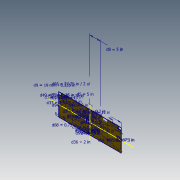
# Autodesk Inventor part: FLUGGER AIR VALVE MTG BRKT
Saved by Autodesk Inventor 2020.3 (Build 243373000, 373)
## iProperties
RuleStatus: InUse
AfterDocSave0: file://Part Number Cleaner
Created: 2019-10-25
Material: ACRYLIC, BLACK
Vendor: HHMI: JRC - ID&F
Document SubType Name: Modeling
Designer: arnoldj
Density: 1 g/cm^3
Appearance: Gold
DESIGN DEPARTMENT: HHMI: JRC - ID&F
ALTERED ITEM PART NUMBER: N/A
ALTERED ITEM VENDOR: N/A
ALTERED ITEM DESCRIPTION: N/A
Author: arnoldj
Revision Number: 0
Autodesk Inventor part; units mm, degrees
ref_plane "YZ Plane" through (0, 0, 0) normal (1, 0, 0) x (0, 1, 0)
ref_plane "XZ Plane" through (0, 0, 0) normal (0, 1, 0) x (-1, 0, 0)
ref_plane "XY Plane" through (0, 0, 0) normal (0, 0, 1) x (1, 0, 0)
sketch "Sketch1" plane through (0, 0, 0) normal (0, 0, 1) x (1, 0, 0)
  line L0 (0, 186.69) -> (0, -186.69) projected
  line L1 (-533.4, 0) -> (533.4, 0) projected
  line L2 (381, -133.35) -> (-381, -133.35)
  line L3 (-381, -133.35) -> (-381, 133.35)
  line L4 (-381, 133.35) -> (381, 133.35)
  line L5 (381, 133.35) -> (381, -133.35)
  line L6 (381, -133.35) -> (-381, 133.35) construction
  line L7 (-381, -133.35) -> (381, 133.35) construction
  line L8 (-170.942, 32.258) -> (-127, 32.258) construction
  line L9 (-127, 32.258) -> (-127, 6.35) construction
  line L10 (-127, 6.35) -> (-170.942, 6.35) construction
  line L11 (-170.942, 6.35) -> (-170.942, 32.258) construction
  line L12 (127, 32.258) -> (170.942, 32.258) construction
  line L13 (170.942, 32.258) -> (170.942, 6.35) construction
  line L14 (170.942, 6.35) -> (127, 6.35) construction
  line L15 (127, 6.35) -> (127, 32.258) construction
  line L16 (-381, 101.6) -> (-346.075, 101.6)
  line L17 (-346.075, 101.6) -> (-346.075, 133.35)
  line L18 (346.075, 133.35) -> (346.075, 101.6)
  line L19 (346.075, 101.6) -> (381, 101.6)
  line L20 (368.3, -114.3) -> (-368.3, -114.3) construction
  line L21 (-368.3, -114.3) -> (-368.3, 82.55) construction
  line L22 (-368.3, 82.55) -> (368.3, 82.55) construction
  line L23 (368.3, 82.55) -> (368.3, -114.3) construction
  line L24 (368.3, -114.3) -> (-368.3, 82.55) construction
  line L25 (-368.3, -114.3) -> (368.3, 82.55) construction
  line L26 (328.6125, -23.8125) -> (357.1875, -23.8125)
  line L27 (357.1875, -23.8125) -> (357.1875, 23.8125)
  line L28 (357.1875, 23.8125) -> (328.6125, 23.8125)
  line L29 (328.6125, 23.8125) -> (328.6125, -23.8125)
  line L30 (328.6125, -23.8125) -> (357.1875, 23.8125) construction
  line L31 (357.1875, -23.8125) -> (328.6125, 23.8125) construction
  line L32 (-42.8625, -23.8125) -> (-14.2875, -23.8125)
  line L33 (-14.2875, -23.8125) -> (-14.2875, 23.8125)
  line L34 (-14.2875, 23.8125) -> (-42.8625, 23.8125)
  line L35 (-42.8625, 23.8125) -> (-42.8625, -23.8125)
  line L36 (-42.8625, -23.8125) -> (-14.2875, 23.8125) construction
  line L37 (-14.2875, -23.8125) -> (-42.8625, 23.8125) construction
  point P0 (0, 0)
  point P1 (-159.004, 6.35)
  point P2 (138.938, 6.35)
  point P3 (-279.4, 122.859)
  point P4 (279.4, 122.859)
  point P5 (-5.08, 122.859)
  point P6 (0, -15.875)
  point P7 (342.9, 0)
  point P8 (-28.575, 0)
  dimension "d0" = 762
  dimension "d1" = 266.7
  dimension "d2" = 43.942
  dimension "d3" = 25.908
  dimension "d4" = 32.004
  dimension "d5" = 127
  dimension "d7" = 32.004
  dimension "d8" = 127
  dimension "d9" = 10.491
  dimension "d65" = 31.75
  dimension "d66" = 346.075
  dimension "d67" = 736.6
  dimension "d68" = 19.05
  dimension "d69" = 19.05
  dimension "d84" = 279.4
  dimension "d85" = 279.4
  dimension "d86" = 5.08
  dimension "d87" = 28.575
  dimension "d88" = 47.625
  dimension "d89" = 0
  dimension "d90" = 28.575
  dimension "d91" = 342.9
  dimension "d94" = 101.092
  constraints: 72 end point, 12 parallel, 10 point on line, 8 coincident, 8 midpoint, 8 perpendicular, 7 horizontal, 5 equal length, 2 horizontal alignment, 1 vertical
  measures "d0" distance of L3.end L4.end
  measures "d1" distance of L2.end L3.end
  measures "d2" distance of L8.start L8.end
  measures "d3" distance of L10.end L8.start
  measures "d4" distance from line of L9 point (-159.004, 6.35)
  measures "d5" distance between parallel lines of L0 L9
  measures "d7" distance from line of L13 point (138.938, 6.35)
  measures "d8" distance between parallel lines of L0 L15
  measures "d9" distance from line of point (-279.4, 122.859) L4
  measures "d65" distance of L16.end L17.end
  measures "d66" distance between parallel lines of L0 L17
  measures "d67" distance of L21.end L22.end
  measures "d68" distance between parallel lines of L20 L2
  measures "d69" distance between parallel lines of L22 L16
  measures "d84" distance from line of L0 point (-279.4, 122.859)
  measures "d85" distance from line of point (279.4, 122.859) L0
  measures "d86" distance from line of L0 point (-5.08, 122.859)
  measures "d87" distance of L33.end L34.end
  measures "d88" distance of L26.end L27.end
  measures "d89" distance from line of point (-28.575, 0) L1
  measures "d90" distance from line of L0 point (-28.575, 0)
  measures "d91" distance from line of point (342.9, 0) L0
  measures "d94" distance from line of point (-170.942, 32.258) L4
extrude "Extrusion1" add sketch "Sketch1" against normal blind 5.842 contours L4 L18 L19 L5 L1 L27 L28 L29 L0 | L0 L1 L33 L34 L35 L3 L16 L17 L4 | L1 L29 L26 L27 L5 L2 L0 | L0 L2 L3 L1 L35 L32 L33 | L33 L32 L35 L1 | L1 L35 L34 L33 | L29 L28 L27 L1 | L1 L27 L26 L29
hole "Hole1" at (-170.942, 32.258, 0) at (-127, 32.258, 0) at (-159.004, 6.35, 0) at (127, 32.258, 0) at (170.942, 32.258, 0) at (138.938, 6.35, 0) direction (0, 0, -1) diameter 3.1242 end through all
thread "Thread1" size "M4x0.7" class "6H" standard "ANSI Metric M Profile" full length
thread "Thread2" size "5-40 UNC" class "2B" standard "ANSI Unified Screw Threads" full length
hole "Hole2" at (-279.4, 122.859, 0) at (279.4, 122.859, 0) at (-5.08, 122.859, 0) direction (0, 0, -1) diameter 6.731 end through all
fillet "Fillet1" radius 9.525 2 edges at (381, -133.35, -2.921) (-381, -133.35, -2.921)
sketch "Sketch2" plane through (0, 0, 0) normal (0, 0, 1) x (1, 0, 0)
  line L0 (0, 118.11) -> (0, -175.26) projected
  line L1 (-520.065, 0) -> (520.065, 0) projected
  line L2 (215.9, -82.55) -> (-215.9, -82.55) construction
  line L3 (-215.9, -82.55) -> (-215.9, 38.1) construction
  line L4 (-215.9, 38.1) -> (215.9, 38.1) construction
  line L5 (215.9, 38.1) -> (215.9, -82.55) construction
  line L6 (215.9, -82.55) -> (-215.9, 38.1) construction
  line L7 (-215.9, -82.55) -> (215.9, 38.1) construction
  line L8 (-371.475, -133.35) -> (371.475, -133.35) construction
  line L9 (-22.86, -121.4084) -> (-22.86, -107.1916) construction
  line L10 (-20.574, -121.4084) -> (-20.574, -107.1916)
  line L11 (-25.146, -107.1916) -> (-25.146, -121.4084)
  arc A0 (-25.146, -121.4084) -> (-20.574, -121.4084) centre (-22.86, -121.4084) ccw
  arc A1 (-20.574, -107.1916) -> (-25.146, -107.1916) centre (-22.86, -107.1916) ccw
  line L12 (-7.62, -121.4084) -> (-7.62, -107.1916) construction
  line L13 (-5.334, -121.4084) -> (-5.334, -107.1916)
  line L14 (-9.906, -107.1916) -> (-9.906, -121.4084)
  arc A2 (-9.906, -121.4084) -> (-5.334, -121.4084) centre (-7.62, -121.4084) ccw
  arc A3 (-5.334, -107.1916) -> (-9.906, -107.1916) centre (-7.62, -107.1916) ccw
  line L15 (-22.86, -114.3) -> (-7.62, -114.3) construction
  point P0 (0, 0)
  point P1 (0, -22.225)
  point P2 (-50.8, -82.55)
  point P3 (50.8, -82.55)
  point P4 (50.8, 38.1)
  point P5 (-50.8, 38.1)
  point P6 (0, -82.55)
  point P7 (0, 38.1)
  point P8 (-215.9, 76.2)
  point P9 (215.9, 76.2)
  point P10 (0, -57.15)
  point P11 (-15.24, -114.3)
  point P12 (-50.8, 76.2)
  point P13 (50.8, 76.2)
  dimension "d35" = 431.8
  dimension "d36" = 50.8
  dimension "d37" = 38.1
  dimension "d38" = 50.8
  dimension "d39" = 50.8
  dimension "d40" = 50.8
  dimension "d41" = 50.8
  dimension "d49" = 76.2
  dimension "d50" = 76.2
  dimension "d96" = 25.4
  dimension "d97" = 2.286
  dimension "d98" = 15.24
  dimension "d99" = 19.05
  dimension "d104" = 7.62
  dimension "d106" = 50.8
  dimension "d107" = 50.8
  constraints: 30 end point, 8 point on circle, 8 tangent, 7 midpoint, 7 point on line, 6 parallel, 4 centre point, 4 coincident, 2 horizontal alignment, 2 perpendicular, 2 vertical alignment, 1 equal radius, 1 horizontal, 1 vertical
  measures "d35" distance of L3.end L4.end
  measures "d36" distance between parallel lines of L2 L8
  measures "d37" distance between parallel lines of L1 L4
  measures "d38" distance from line of L0 point (-50.8, 38.1)
  measures "d39" distance from line of L0 point (50.8, 38.1)
  measures "d40" distance from line of L0 point (-50.8, -82.55)
  measures "d41" distance from line of L0 point (50.8, -82.55)
  measures "d49" distance from line of L1 point (-215.9, 76.2)
  measures "d50" distance from line of L1 point (215.9, 76.2)
  measures "d96" distance of point (0, -82.55) point (0, -57.15)
  measures "d97" radius of A1
  measures "d98" distance between parallel lines of L12 L9
  measures "d99" distance from line of L8 L15.start
  measures "d104" distance between parallel lines of L0 L12
  measures "d106" distance from line of L0 point (-50.8, 76.2)
  measures "d107" distance from line of point (50.8, 76.2) L0
hole "Hole3" at (-215.9, 38.1, 0) at (-50.8, 38.1, 0) at (0, 38.1, 0) at (50.8, 38.1, 0) at (215.9, 38.1, 0) at (215.9, -82.55, 0) at (50.8, -82.55, 0) at (-50.8, -82.55, 0) at (-215.9, -82.55, 0) at (-215.9, 76.2, 0) at (215.9, 76.2, 0) at (0, -57.15, 0) at (-50.8, 76.2, 0) at (50.8, 76.2, 0) direction (0, 0, -1) diameter 3.1242 end through all
sketch "Sketch3" plane through (0, 0, 0) normal (0, 0, 1) x (1, 0, 0)
  line L0 (0, 176.8424) -> (0, -127.6045) projected
  line L1 (-484.505, 0) -> (484.505, 0) projected
  circle A0 centre (-215.9, -82.55) radius 1.5621 projected
  line L2 (346.075, 133.35) -> (-346.075, 133.35) projected
  point P0 (0, 0)
  point P1 (-254, -59.69)
  point P2 (-254, -25.4)
  dimension "d51" = 34.29
  dimension "d52" = 0
  dimension "d53" = 254
  dimension "d54" = 25.4
  dimension "d95" = 158.75
  measures "d51" distance of point (-254, -59.69) point (-254, -25.4)
  measures "d52" horizontal distance of point (-254, -25.4) point (-254, -59.69)
  measures "d53" distance from line of L0 point (-254, -25.4)
  measures "d54" distance from line of point (-254, -25.4) L1
  measures "d95" distance from line of point (-254, -25.4) L2
hole "Hole4" at (-254, -25.4, 0) at (-254, -59.69, 0) direction (0, 0, -1) diameter 3.1242 end through all
pattern_linear "Rectangular Pattern1" count 2 spacing 508 along (1, 0, 0) of "Hole4"
hole "Hole5" at (368.3, -114.3, 0) at (368.3, 82.55, 0) at (-368.3, 82.55, 0) at (-368.3, -114.3, 0) direction (0, 0, -1) diameter 7.0104 end through all clearance for "Socket Head Cap Screw" size "M6" standard "Ansi Metric M Profile"
fillet "Fillet2" radius 3.175 6 edges at (-381, 101.6, -2.921) (-346.075, 101.6, -2.921) (-346.075, 133.35, -2.921) (346.075, 133.35, -2.921) (381, 101.6, -2.921) (346.075, 101.6, -2.921)
sketch "Sketch4" plane through (0, 0, 0) normal (0, 0, 1) x (1, 0, 0)
  line L0 (342.9, 133.35) -> (-342.9, 133.35) projected
  line L1 (212.3694, 97.79) -> (156.4894, 97.79)
  line L2 (156.4894, 97.79) -> (156.4894, 133.35)
  line L3 (156.4894, 133.35) -> (212.3694, 133.35)
  line L4 (212.3694, 133.35) -> (212.3694, 97.79)
  line L5 (212.3694, 97.79) -> (156.4894, 133.35) construction
  line L6 (156.4894, 97.79) -> (212.3694, 133.35) construction
  line L7 (0, 186.69) -> (0, -186.69) projected
  point P0 (0, 0)
  point P1 (184.4294, 115.57)
  point P2 (212.3694, 133.35)
  dimension "d78" = 55.88
  dimension "d80" = 35.56
  dimension "d83" = 184.4294
  constraints: 12 end point, 2 midpoint, 2 parallel, 1 horizontal, 1 perpendicular, 1 point on line
  measures "d78" distance of L1.start L1.end
  measures "d80" distance of L1.end L2.end
  measures "d83" distance from line of point (184.429, 115.57) L7
extrude "Extrusion2" cut sketch "Sketch4" against normal through all
extrude "Extrusion3" [suppressed]
extrude "Extrusion4" cut sketch "Sketch2" against normal through all
mirror "Mirror2" about plane through (0, 0, 0) normal (1, 0, 0) of "Extrusion4"
fillet "Fillet3" radius 3.175 4 edges at (156.4894, 133.35, -2.921) (156.4894, 97.79, -2.921) (212.3694, 97.79, -2.921) (212.3694, 133.35, -2.921)
body "Solid1"
